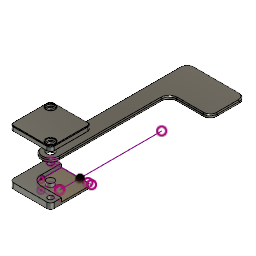
Mailbox_Flag (Autodesk Fusion 360 design; units mm, degrees)
Autodesk Fusion 360 part; units mm, degrees
note: some values were not read from the file. Set by a fixed rule: which sketch regions a step uses.
sketch "Sketch1" plane through (0, 0, 0) normal (0, 0, 1) x (1, 0, 0) in component "Component"
  line L0 (0, 0) -> (45, 0) construction
  line L1 (45, 0) -> (45, 45) construction
  line L2 (45, 45) -> (0, 45) construction
  line L3 (0, 45) -> (0, 0) construction
  line L4 (0, 45) -> (45, 0) construction
  line L5 (0, 0) -> (45, 45) construction
  circle A0 centre (22.5, 22.5) radius 10
  line L6 (12.5, 22.5) -> (12.5, 45)
  line L7 (22.5, 12.5) -> (45, 12.5)
  circle A1 centre (22.5, 22.5) radius 4
  line L8 (32.5, 22.5) -> (32.5, 45) construction
  line L9 (12.5, 45) -> (0, 32.5) construction
  line L10 (45, 12.5) -> (32.5, 0) construction
  circle A2 centre (6.25, 38.75) radius 2.95
  circle A3 centre (6.25, 38.75) radius 4.45
  circle A4 centre (38.75, 6.25) radius 2.95
  circle A5 centre (38.75, 6.25) radius 4.45
  line L11 (0, 41) -> (0, 4)
  line L12 (4, 0) -> (41, 0)
  line L13 (45, 4) -> (45, 41)
  line L14 (41, 45) -> (4, 45)
  arc A6 (4, 45) -> (0, 41) centre (4, 41) ccw
  arc A7 (45, 41) -> (41, 45) centre (41, 41) ccw
  arc A8 (41, 0) -> (45, 4) centre (41, 4) ccw
  arc A9 (0, 4) -> (4, 0) centre (4, 4) ccw
  circle A10 centre (22.5, 22.5) radius 4.4
  line L15 (12.1, 22.5) -> (12.1, 45)
  circle A11 centre (22.5, 22.5) radius 10.4
  line L16 (22.5, 12.1) -> (45, 12.1)
  dimension "d1" = 45
  dimension "d2" = 45
  dimension "d5" = 20
  dimension "d6" = 8
  dimension "d24" = 5.9
  dimension "d25" = 8.9
  dimension "d26" = 5.9
  dimension "d27" = 8.9
  dimension "d30" = 4
  dimension "d31" = 4
  dimension "d32" = 4
  dimension "d33" = 4
  dimension "d69" = 0.4
  dimension "d70" = 0.4
  dimension "d71" = 0.4
  dimension "d72" = 0.4
  measures "d5" diameter of A0
  measures "d6" diameter of A1
  measures "d24" diameter of A2
  measures "d25" diameter of A3
  measures "d26" diameter of A4
  measures "d27" diameter of A5
  measures "d30" radius of A6
  measures "d31" radius of A7
  measures "d32" radius of A8
  measures "d33" radius of A9
  measures "d70" distance of L6
  measures "d72" distance of L7
extrude "Extrude5" add sketch "Sketch1" along normal blind 2.4 contours A0 | A0 L6 L7 A11 | A0 L6 L7 A11 | L6 L14 L15 A11 | L6 L7 L13 L14 A7 A11 | L7 L13 A11 L16 | A10 makes body 1 in component "Component"
extrude "Extrude7" add sketch "Sketch1" along normal blind 6.4 contours L11 L12 L13 L14 A6 A8 A9 L15 A11 L16 | A1 | A3 | A5 bodies 1 in component "Component"
ref_plane "WorkPlane2" through (0, 0, 60) normal (0, 0, 1) x (1, 0, 0) in component "Component"
sketch "Sketch3" plane through (0, 0, 60) normal (0, 0, 1) x (1, 0, 0) in component "Component"
  line L0 (4, 0) -> (41, 0)
  arc A0 (41, 0) -> (45, 4) centre (41, 4) ccw
  line L1 (45, 4) -> (45, 41)
  arc A1 (45, 41) -> (41, 45) centre (41, 41) ccw
  line L2 (41, 45) -> (4, 45)
  arc A2 (4, 45) -> (0, 41) centre (4, 41) ccw
  line L3 (0, 41) -> (0, 4)
  arc A3 (0, 4) -> (4, 0) centre (4, 4) ccw
  circle A4 centre (6.25, 38.75) radius 4.45
  circle A5 centre (6.25, 38.75) radius 2.95
  circle A6 centre (22.5, 22.5) radius 4
  circle A7 centre (38.75, 6.25) radius 4.45
  circle A8 centre (38.75, 6.25) radius 2.95
  circle A9 centre (22.5, 22.5) radius 4.4
extrude "Extrude8" add sketch "Sketch3" against normal blind 2.4 separate body contours L0 A0 L1 A1 L2 A2 L3 A3 | A4 | A6 | A7 | A9 makes body 2 in component "Component"
extrude "Extrude9" add sketch "Sketch3" against normal blind 4.8 contours L0 A0 L1 A1 L2 A2 L3 A3 | A4 | A6 | A7 | A9 bodies 2 in component "Component"
extrude "Extrude10" cut sketch "Sketch3" against normal blind 2.4 contours A4 | A7 bodies 2 in component "Component"
ref_plane "WorkPlane3" through (0, 0, 30) normal (0, 0, 1) x (1, 0, 0) in component "Component"
sketch "Sketch4" plane through (0, 0, 30) normal (0, 0, 1) x (1, 0, 0) in component "Component"
  circle A0 centre (22.5, 22.5) radius 10
  circle A1 centre (22.5, 22.5) radius 4
  line L0 (0, 0) -> (45, 45)
  line L1 (45, 45) -> (0, 45)
  line L2 (12.5, 12.5) -> (12.5, 182.5) construction
  line L3 (0, 45) -> (45, 0)
  line L4 (22.5, 12.5) -> (45, 12.5)
  line L5 (32.5, 22.5) -> (32.5, 45)
  line L6 (32.5, 12.5) -> (32.5, 142.5) construction
  line L7 (12.5, 182.5) -> (77.5, 182.5) construction
  line L8 (12.5, 22.5) -> (12.5, 45)
  line L9 (77.5, 182.5) -> (77.5, 142.5) construction
  line L10 (77.5, 142.5) -> (32.5, 142.5) construction
  line L11 (12.5, 12.5) -> (12.5, 174.5)
  line L12 (20.5, 182.5) -> (69.5, 182.5)
  line L13 (77.5, 174.5) -> (77.5, 150.5)
  line L14 (69.5, 142.5) -> (40.5, 142.5)
  line L15 (32.5, 134.5) -> (32.5, 12.5)
  arc A2 (20.5, 182.5) -> (12.5, 174.5) centre (20.5, 174.5) ccw
  arc A3 (77.5, 174.5) -> (69.5, 182.5) centre (69.5, 174.5) ccw
  arc A4 (69.5, 142.5) -> (77.5, 150.5) centre (69.5, 150.5) ccw
  arc A5 (40.5, 142.5) -> (32.5, 134.5) centre (40.5, 134.5) ccw
  circle A6 centre (22.5, 22.5) radius 4.4
  dimension "d48" = 170
  dimension "d49" = 130
  dimension "d50" = 65
  dimension "d51" = 40
  dimension "d52" = 8
  dimension "d53" = 8
  dimension "d54" = 8
  dimension "d55" = 8
  measures "d49" distance of L0.start
  measures "d50" distance of L0.start
  measures "d52" radius of A2
  measures "d53" radius of A3
  measures "d54" radius of A4
  measures "d55" radius of A5
extrude "Extrude11" add sketch "Sketch4" along normal blind 4 separate body contours A0 L0 L3 A6 | A0 L0 L5 L15 | A0 L0 L3 A6 | A0 L0 L1 L3 L5 L8 L11 L15 | A0 L0 L3 A6 | A0 L0 L3 A6 | A0 L3 L8 L11 | L1 L11 L12 L13 L14 L15 A2 A3 A4 A5 makes body 3 in component "Component"
sketch "Sketch5" plane through (0, 0, 2.4) normal (0, 0, 1) x (-1, 0, 0) in component "Component"
  line L0 (-45, -12.1) -> (-45, -41)
  arc A0 (-45, -41) -> (-41, -45) centre (-41, -41) ccw
  line L1 (-41, -45) -> (-12.1, -45)
  line L2 (-32.5, -22.5) -> (-32.5, -45)
  line L3 (-45, -45) -> (0, -45)
  line L4 (-32.5, -22.5) -> (-32.5, -134.5)
  line L5 (-41, -45) -> (-4, -45)
  arc A1 (-12.1, -22.5) -> (-22.5, -12.1) centre (-22.5, -22.5) ccw
  line L6 (-22.5, -12.1) -> (-45, -12.1)
  line L7 (-12.1, -45) -> (-12.1, -22.5)
  circle A2 centre (-22.5, -22.5) radius 4
  line L8 (-32.5, -45) -> (-32.9, -45) construction
  line L9 (-32.9, -45) -> (-32.9, -43.8) construction
  line L10 (-32.9, -43.8) -> (-32.5, -43.8) construction
  line L11 (-32.5, -43.8) -> (-32.5, -45) construction
  line L12 (-32.9, -43.8) -> (-34.4, -43.8) construction
  line L13 (-34.4, -43.8) -> (-34.4, -42.6) construction
  line L14 (-34.4, -42.6) -> (-32.9, -42.6) construction
  line L15 (-32.9, -42.6) -> (-32.9, -43.8) construction
  circle A3 centre (-33.65, -43.05) radius 0.75
  dimension "d75" = 0.4
  dimension "d76" = 1.2
  dimension "d77" = 1.5
  dimension "d78" = 1.2
  dimension "d79" = 0.75
  measures "d79" radius of A3
chamfer "Chamfer1" distance 0.6 angle 45 2 edges at (2.1011, 40.3592, 60) (34.6011, 7.8592, 60) on bodies 2 in component "Component"
chamfer "Chamfer2" distance 0.6 angle 45 8 edges at (1.1716, 1.1716, 60) (22.5, 0, 60) (43.8284, 1.1716, 60) (45, 22.5, 60) (43.8284, 43.8284, 60) (22.5, 45, 60) (1.1716, 43.8284, 60) (0, 22.5, 60) on bodies 2 in component "Component"
chamfer "Chamfer3" distance 1 angle 45 20 edges at (32.5, 78.5, 34) (34.8431, 140.1569, 34) (55, 142.5, 34) (75.1569, 144.8431, 34) (77.5, 162.5, 34) (75.1569, 180.1569, 34) (45, 182.5, 34) (14.8431, 180.1569, 34) (12.5, 98.5, 34) (22.5, 12.5, 34) (14.8431, 180.1569, 30) (45, 182.5, 30) (75.1569, 180.1569, 30) (77.5, 162.5, 30) (75.1569, 144.8431, 30) (55, 142.5, 30) (34.8431, 140.1569, 30) (32.5, 78.5, 30) (22.5, 12.5, 30) (12.5, 98.5, 30) on bodies 3 in component "Component"
extrude "Extrude13" add sketch "Sketch5" along normal blind 0.4 contours A3 bodies 1 in component "Component"
component "Component" placed x (1, 0, 0) y (0, 1, 0) z (0, 0, 1) at (0, 0, 0)
equation "d1 = BaseSize"
equation "d2 = BaseSize"
equation "HoleDiameter = 8 mm"
equation "ArmWidth = 20 mm"
equation "d5 = ArmWidth"
equation "d6 = HoleDiameter"
equation "PlateThickness = 2.4 mm"
equation "ArmThickness = 4 mm"
equation "PrintingTolerance = 0.2 mm"
equation "ArmLength = 170 mm"
equation "FlagHeight = 40 mm"
equation "FlagWidth = 65 mm"
equation "ScrewDiameter = 5.5 mm"
equation "ScrewHeadDiameter = 8.5 mm"
equation "BaseSize = 45 mm"
equation "d24 = ScrewDiameter + PrintingTolerance * 2"
equation "d25 = ScrewHeadDiameter + PrintingTolerance * 2"
equation "d26 = ScrewDiameter + PrintingTolerance * 2"
equation "d27 = ScrewHeadDiameter + PrintingTolerance * 2"
equation "d30 = MountFilletRadius"
equation "d31 = MountFilletRadius"
equation "d32 = MountFilletRadius"
equation "d33 = MountFilletRadius"
equation "d34 = PlateThickness"
equation "d38 = PlateThickness + ArmThickness"
equation "d41 = -PlateThickness"
equation "d43 = -( PlateThickness * 2 )"
equation "d45 = -PlateThickness"
equation "d48 = ArmLength"
equation "d49 = ArmLength - FlagHeight"
equation "d50 = FlagWidth"
equation "d51 = FlagHeight"
equation "d56 = ArmThickness"
equation "NubThickness = 0.4 mm"
equation "d69 = PrintingTolerance * 2"
equation "d70 = PrintingTolerance * 2"
equation "d71 = PrintingTolerance * 2"
equation "d72 = PrintingTolerance * 2"
equation "d75 = PrintingTolerance * 2"
equation "d79 = d77 / 2"
equation "MountFilletRadius = 4 mm"
named bodies: "Mount Bottom", "Mount Top", "Flag"
